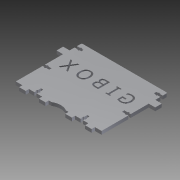
# Autodesk Inventor part: suport z darrera
Saved by Autodesk Inventor 2012 SP1 (Build 160190100, 190)
## iProperties
Created: 2015-03-29
Part Number: suport z darrera
Material: Default
Document SubType Name: Modeling
Designer: sheina
Density: 1 g/cm^3
Author: sheina
Autodesk Inventor part; units mm, degrees
ref_plane "YZ Plane" through (0, 0, 0) normal (1, 0, 0) x (0, 1, 0)
ref_plane "XZ Plane" through (0, 0, 0) normal (0, 1, 0) x (-1, 0, 0)
ref_plane "XY Plane" through (0, 0, 0) normal (0, 0, 1) x (1, 0, 0)
sketch "Boceto1" plane through (0, 0, 0) normal (0, 0, 1) x (1, 0, 0)
  line L0 (130, 0) -> (130, 95)
  line L1 (0, 95) -> (0, 0)
  line L2 (20, 0) -> (20, -5)
  line L3 (10, -5) -> (10, 0)
  line L4 (50, 0) -> (50, -5)
  line L5 (40, -5) -> (40, 0)
  line L6 (90, 0) -> (90, -5)
  line L7 (80, -5) -> (80, 0)
  line L8 (120, 0) -> (120, -5)
  line L9 (110, -5) -> (110, 0)
  line L10 (20, -5) -> (10, -5)
  line L11 (50, -5) -> (40, -5)
  line L12 (0, 0) -> (10, 0)
  line L13 (20, 0) -> (40, 0)
  line L14 (120, -5) -> (110, -5)
  line L15 (90, -5) -> (80, -5)
  line L16 (50, 0) -> (80, 0)
  line L17 (90, 0) -> (110, 0)
  line L18 (120, 0) -> (130, 0)
  line L19 (130, 100) -> (0, 100)
  line L20 (0, 95) -> (0, 100)
  line L21 (130, 95) -> (130, 100)
  dimension "d0" = 130
  dimension "d5" = 10
  dimension "d6" = 10
  dimension "d7" = 10
  dimension "d8" = 10
  dimension "d9" = 10
  dimension "d10" = 10
  dimension "d11" = 20
  dimension "d12" = 20
  constraints: 44 end point, 10 perpendicular, 7 parallel, 5 horizontal
  measures "d0" distance between parallel lines of L0 L1
  measures "d5" distance between parallel lines of L3 L2
  measures "d6" distance between parallel lines of L4 L5
  measures "d7" distance between parallel lines of L6 L7
  measures "d8" distance between parallel lines of L9 L8
  measures "d9" distance between parallel lines of L3 L1
  measures "d10" distance between parallel lines of L0 L8
  measures "d11" distance between parallel lines of L6 L9
  measures "d12" distance between parallel lines of L5 L2
extrude "Extrusión1" add sketch "Boceto1" along normal blind 5
sketch "Boceto2" plane through (0, 0, 5) normal (0, 0, 1) x (1, 0, 0)
  line L0 (80, 0) -> (50, 0) projected
  arc A0 (75.8724, 0) -> (54.3573, 0) centre (65.1148, -17.6132) ccw
  constraints: 2 point on circle, 2 point on line, 1 centre point
extrude "Extrusión2" cut sketch "Boceto2" against normal blind 5
sketch "Boceto3" plane through (0, 0, 5) normal (0, 0, 1) x (1, 0, 0)
  line L0 (80, -5) -> (80, 0) projected
  line L1 (40, 0) -> (20, 0) projected
  line L2 (98.3739, -0.0977) -> (98.3739, 2.6763)
  line L3 (98.3739, 2.6763) -> (97.3739, 2.6763)
  line L4 (97.3739, 2.6763) -> (97.3739, 5.0763)
  line L5 (97.3739, 5.0763) -> (98.3739, 5.0763)
  line L6 (98.3739, 5.0763) -> (98.3739, 9.9876)
  line L7 (98.3739, 9.9876) -> (101.8739, 9.9876)
  line L8 (101.8739, 9.9876) -> (101.8739, 5.0763)
  line L9 (101.8739, 5.0763) -> (102.8739, 5.0763)
  line L10 (102.8739, 5.0763) -> (102.8739, 2.6763)
  line L11 (102.8739, 2.6763) -> (101.8739, 2.6763)
  line L12 (101.8739, 2.6763) -> (101.8739, -0.0977)
  line L13 (28.1584, 5.0695) -> (28.1584, 9.9808)
  line L14 (31.6584, 9.9808) -> (31.6584, 5.0695)
  line L15 (28.1584, 9.9808) -> (31.6584, 9.9808)
  line L16 (27.1584, 5.0695) -> (28.1584, 5.0695)
  line L17 (28.1584, 2.6695) -> (27.1584, 2.6695)
  line L18 (27.1584, 2.6695) -> (27.1584, 5.0695)
  line L19 (31.6584, 2.6695) -> (31.6584, -0.1046)
  line L20 (28.1584, -0.1046) -> (28.1584, 2.6695)
  line L21 (32.6584, 2.6695) -> (31.6584, 2.6695)
  line L22 (32.6584, 5.0695) -> (32.6584, 2.6695)
  line L23 (31.6584, 5.0695) -> (32.6584, 5.0695)
  line L24 (28.1584, -0.1046) -> (31.6584, -0.1046)
  line L25 (98.3739, -0.0977) -> (101.8739, -0.0977)
  dimension "d18" = 3.5
  constraints: 48 end point, 3 parallel
  measures "d18" distance between parallel lines of L19 L20
extrude "Extrusión3" cut sketch "Boceto3" against normal blind 5
fillet "Empalme1" radius 2 2 edges at (130, 100, 2.5) (0, 100, 2.5)
sketch "Boceto5" plane through (0, 0, 0) normal (0, 0, -1) x (-1, 0, 0)
  line L0 (-115.5606, 70.7599) -> (-4.4465, 70.7599) construction
  line L1 (-4.4465, 70.7599) -> (-4.4465, 16.0729) construction
  line L2 (-4.4465, 16.0729) -> (-115.5606, 16.0729) construction
  line L3 (-115.5606, 16.0729) -> (-115.5606, 70.7599) construction
  spline S0 degree 2 poles (-106.196, 52.0306) (-108.1068, 52.0306) (-111.2721, 53.1975) (-112.4099, 54.379) knots 0 0 0 1 2 2 2
  spline S1 degree 2 poles (-112.4099, 54.379) (-113.5477, 55.5751) (-114.7584, 59.1051) (-114.7584, 61.3952) knots 0 0 0 1 2 2 2
  spline S2 degree 2 poles (-114.7584, 61.3952) (-114.7584, 63.5687) (-113.5331, 67.0111) (-112.3953, 68.2364) knots 0 0 0 1 2 2 2
  spline S3 degree 2 poles (-112.3953, 68.2364) (-111.3013, 69.4179) (-108.0922, 70.7016) (-106.1814, 70.7016) knots 0 0 0 1 2 2 2
  spline S4 degree 2 poles (-106.1814, 70.7016) (-105.2624, 70.7016) (-103.5995, 70.439) (-102.841, 70.2056) knots 0 0 0 1 2 2 2
  spline S5 degree 2 poles (-102.841, 70.2056) (-102.2284, 70.0306) (-100.7405, 69.3888) (-100.2884, 69.1554) knots 0 0 0 1 2 2 2
  line L4 (-100.2884, 69.1554) -> (-100.2884, 66.2672)
  line L5 (-100.2884, 66.2672) -> (-100.4926, 66.2672)
  spline S6 degree 2 poles (-100.4926, 66.2672) (-100.9448, 66.661) (-101.8929, 67.3758) (-102.7681, 67.7842) knots 0 0 0 1 2 2 2
  spline S7 degree 2 poles (-102.7681, 67.7842) (-103.4974, 68.1489) (-105.3791, 68.6302) (-106.4585, 68.6302) knots 0 0 0 1 2 2 2
  spline S8 degree 2 poles (-106.4585, 68.6302) (-109.055, 68.6302) (-112.264, 64.721) (-112.264, 61.4682) knots 0 0 0 1 2 2 2
  spline S9 degree 2 poles (-112.264, 61.4682) (-112.264, 59.6594) (-111.418, 56.9463) (-110.6157, 56.0127) knots 0 0 0 1 2 2 2
  spline S10 degree 2 poles (-110.6157, 56.0127) (-109.8427, 55.0792) (-107.6546, 54.1019) (-106.2835, 54.1019) knots 0 0 0 1 2 2 2
  spline S11 degree 2 poles (-106.2835, 54.1019) (-105.277, 54.1019) (-103.264, 54.3936) (-102.5785, 54.6853) knots 0 0 0 1 2 2 2
  line L6 (-102.5785, 54.6853) -> (-102.5785, 59.3385)
  line L7 (-102.5785, 59.3385) -> (-106.7503, 59.3385)
  line L8 (-106.7503, 59.3385) -> (-106.7503, 61.439)
  line L9 (-106.7503, 61.439) -> (-100.2154, 61.439)
  line L10 (-100.2154, 61.439) -> (-100.2154, 53.5768)
  spline S12 degree 2 poles (-100.2154, 53.5768) (-100.6676, 53.3725) (-102.2138, 52.7453) (-102.8702, 52.5557) knots 0 0 0 1 2 2 2
  spline S13 degree 2 poles (-102.8702, 52.5557) (-103.76, 52.2931) (-105.1895, 52.0306) (-106.196, 52.0306) knots 0 0 0 1 2 2 2
  line L11 (-83.2073, 52.3806) -> (-90.1798, 52.3806)
  line L12 (-90.1798, 52.3806) -> (-90.1798, 54.2186)
  line L13 (-90.1798, 54.2186) -> (-87.8897, 54.2186)
  line L14 (-87.8897, 54.2186) -> (-87.8897, 68.5427)
  line L15 (-87.8897, 68.5427) -> (-90.1798, 68.5427)
  line L16 (-90.1798, 68.5427) -> (-90.1798, 70.3806)
  line L17 (-90.1798, 70.3806) -> (-83.2073, 70.3806)
  line L18 (-83.2073, 70.3806) -> (-83.2073, 68.5427)
  line L19 (-83.2073, 68.5427) -> (-85.4974, 68.5427)
  line L20 (-85.4974, 68.5427) -> (-85.4974, 54.2186)
  line L21 (-85.4974, 54.2186) -> (-83.2073, 54.2186)
  line L22 (-83.2073, 54.2186) -> (-83.2073, 52.3806)
  spline S14 degree 2 poles (-60.3062, 57.909) (-60.3062, 56.567) (-61.3273, 54.5103) (-62.1733, 53.8393) knots 0 0 0 1 2 2 2
  spline S15 degree 2 poles (-62.1733, 53.8393) (-63.1944, 53.0516) (-65.5136, 52.3806) (-67.3516, 52.3806) knots 0 0 0 1 2 2 2
  line L23 (-67.3516, 52.3806) -> (-72.5153, 52.3806)
  line L24 (-72.5153, 52.3806) -> (-72.5153, 70.3806)
  line L25 (-72.5153, 70.3806) -> (-67.7454, 70.3806)
  spline S16 degree 2 poles (-67.7454, 70.3806) (-65.82, 70.3806) (-63.8945, 70.1327) (-63.0193, 69.6513) knots 0 0 0 1 2 2 2
  spline S17 degree 2 poles (-63.0193, 69.6513) (-62.042, 69.1408) (-61.1522, 67.4633) (-61.1522, 66.3255) knots 0 0 0 1 2 2 2
  spline S18 degree 2 poles (-61.1522, 66.3255) (-61.1522, 65.0565) (-62.4942, 63.0435) (-63.6757, 62.4747) knots 0 0 0 1 2 2 2
  line L26 (-63.6757, 62.4747) -> (-63.6757, 62.3871)
  spline S19 degree 2 poles (-63.6757, 62.3871) (-62.0712, 61.9495) (-60.3062, 59.6302) (-60.3062, 57.909) knots 0 0 0 1 2 2 2
  spline S20 degree 2 poles (-62.8005, 57.8069) (-62.8005, 58.828) (-63.384, 60.1408) (-64.2592, 60.6076) knots 0 0 0 1 2 2 2
  spline S21 degree 2 poles (-64.2592, 60.6076) (-64.8281, 60.8993) (-66.17, 61.0743) (-67.4099, 61.0743) knots 0 0 0 1 2 2 2
  line L27 (-67.4099, 61.0743) -> (-70.123, 61.0743)
  line L28 (-70.123, 61.0743) -> (-70.123, 54.4228)
  line L29 (-70.123, 54.4228) -> (-68.183, 54.4228)
  spline S22 degree 2 poles (-68.183, 54.4228) (-66.6076, 54.4228) (-64.7989, 54.7145) (-64.0987, 55.1813) knots 0 0 0 1 2 2 2
  spline S23 degree 2 poles (-64.0987, 55.1813) (-63.4277, 55.6627) (-62.8005, 56.8588) (-62.8005, 57.8069) knots 0 0 0 1 2 2 2
  spline S24 degree 2 poles (-63.6465, 65.99) (-63.6465, 66.6319) (-64.0841, 67.5946) (-64.5655, 67.8717) knots 0 0 0 1 2 2 2
  spline S25 degree 2 poles (-64.5655, 67.8717) (-65.149, 68.1926) (-66.5639, 68.3385) (-67.8329, 68.3385) knots 0 0 0 1 2 2 2
  line L30 (-67.8329, 68.3385) -> (-70.123, 68.3385)
  line L31 (-70.123, 68.3385) -> (-70.123, 63.0727)
  line L32 (-70.123, 63.0727) -> (-67.4099, 63.0727)
  spline S26 degree 2 poles (-67.4099, 63.0727) (-66.2867, 63.0727) (-65.2219, 63.3061) (-64.653, 63.6708) knots 0 0 0 1 2 2 2
  spline S27 degree 2 poles (-64.653, 63.6708) (-64.0987, 64.0208) (-63.6465, 65.144) (-63.6465, 65.99) knots 0 0 0 1 2 2 2
  spline S28 degree 2 poles (-37.4634, 68.3239) (-36.4423, 67.1278) (-35.3046, 63.627) (-35.3046, 61.3806) knots 0 0 0 1 2 2 2
  spline S29 degree 2 poles (-35.3046, 61.3806) (-35.3046, 59.1926) (-36.4132, 55.6481) (-37.4634, 54.452) knots 0 0 0 1 2 2 2
  spline S30 degree 2 poles (-37.4634, 54.452) (-38.572, 53.1975) (-41.5039, 52.0014) (-43.2689, 52.0014) knots 0 0 0 1 2 2 2
  spline S31 degree 2 poles (-43.2689, 52.0014) (-45.0922, 52.0014) (-48.0096, 53.2413) (-49.0744, 54.452) knots 0 0 0 1 2 2 2
  spline S32 degree 2 poles (-49.0744, 54.452) (-50.1101, 55.6481) (-51.2187, 59.1635) (-51.2187, 61.3806) knots 0 0 0 1 2 2 2
  spline S33 degree 2 poles (-51.2187, 61.3806) (-51.2187, 63.6416) (-50.0955, 67.0841) (-49.0598, 68.3239) knots 0 0 0 1 2 2 2
  spline S34 degree 2 poles (-49.0598, 68.3239) (-48.0096, 69.52) (-45.0777, 70.7599) (-43.2689, 70.7599) knots 0 0 0 1 2 2 2
  spline S35 degree 2 poles (-43.2689, 70.7599) (-41.431, 70.7599) (-38.4845, 69.4763) (-37.4634, 68.3239) knots 0 0 0 1 2 2 2
  spline S36 degree 2 poles (-37.7989, 61.3806) (-37.7989, 63.1602) (-38.572, 65.9171) (-39.2721, 66.8215) knots 0 0 0 1 2 2 2
  spline S37 degree 2 poles (-39.2721, 66.8215) (-39.9869, 67.755) (-41.9999, 68.6886) (-43.2543, 68.6886) knots 0 0 0 1 2 2 2
  spline S38 degree 2 poles (-43.2543, 68.6886) (-44.5525, 68.6886) (-46.5072, 67.7842) (-47.2511, 66.8215) knots 0 0 0 1 2 2 2
  spline S39 degree 2 poles (-47.2511, 66.8215) (-47.9658, 65.9025) (-48.7243, 63.1311) (-48.7243, 61.3806) knots 0 0 0 1 2 2 2
  spline S40 degree 2 poles (-48.7243, 61.3806) (-48.7243, 57.8361) (-45.7486, 54.0727) (-43.2543, 54.0727) knots 0 0 0 1 2 2 2
  spline S41 degree 2 poles (-43.2543, 54.0727) (-40.76, 54.0727) (-37.7989, 57.8361) (-37.7989, 61.3806) knots 0 0 0 1 2 2 2
  line L33 (-12.5055, 52.3806) -> (-15.2478, 52.3806)
  line L34 (-15.2478, 52.3806) -> (-19.6239, 59.5573)
  line L35 (-19.6239, 59.5573) -> (-24.0874, 52.3806)
  line L36 (-24.0874, 52.3806) -> (-26.6692, 52.3806)
  line L37 (-26.6692, 52.3806) -> (-20.9367, 61.3952)
  line L38 (-20.9367, 61.3952) -> (-26.4942, 70.3806)
  line L39 (-26.4942, 70.3806) -> (-23.7519, 70.3806)
  line L40 (-23.7519, 70.3806) -> (-19.4634, 63.3353)
  line L41 (-19.4634, 63.3353) -> (-15.0874, 70.3806)
  line L42 (-15.0874, 70.3806) -> (-12.5055, 70.3806)
  line L43 (-12.5055, 70.3806) -> (-18.136, 61.5119)
  line L44 (-18.136, 61.5119) -> (-12.5055, 52.3806)
  constraints: 2 other
extrude "Extrusión5" cut sketch "Boceto5" against normal blind 10
sketch "Boceto6" plane through (0, 0, 5) normal (0, 0, 1) x (1, 0, 0)
  line L0 (0, 0) -> (0, 100) projected
  line L1 (130, 100) -> (130, 0) projected
  line L2 (-9.8, 81.57) -> (-9.8, 71.57)
  line L3 (139.8, 71.57) -> (139.8, 81.57)
  line L4 (0, 71.57) -> (0, 81.57)
  line L5 (130, 81.57) -> (130, 71.57)
  line L6 (139.8, 81.57) -> (130, 81.57)
  line L7 (0, 81.57) -> (-9.8, 81.57)
  line L8 (-9.8, 71.57) -> (0, 71.57)
  line L9 (130, 71.57) -> (139.8, 71.57)
  point P0 (130, 93)
  point P1 (0, 93)
  dimension "d27" = 9.8
  dimension "d28" = 9.8
  constraints: 16 end point, 5 parallel, 4 point on line, 2 horizontal, 2 perpendicular
  measures "d27" distance between parallel lines of L0 L2
  measures "d28" distance between parallel lines of L1 L3
extrude "Extrusión6" add sketch "Boceto6" against normal blind 5
sketch "Boceto7" plane through (0, 0, 5) normal (0, 0, 1) x (1, 0, 0)
  line L0 (0, 0) -> (0, 71.57) projected
  line L1 (130.2524, 40.7442) -> (127.5829, 40.7442)
  line L2 (127.5829, 40.7442) -> (127.5829, 39.7442)
  line L3 (127.5829, 39.7442) -> (125.1829, 39.7442)
  line L4 (125.1829, 39.7442) -> (125.1829, 40.7442)
  line L5 (125.1829, 40.7442) -> (120.2716, 40.7442)
  line L6 (120.2716, 40.7442) -> (120.2716, 44.2442)
  line L7 (120.2716, 44.2442) -> (125.1829, 44.2442)
  line L8 (125.1829, 44.2442) -> (125.1829, 45.2442)
  line L9 (125.1829, 45.2442) -> (127.5829, 45.2442)
  line L10 (127.5829, 45.2442) -> (127.5829, 44.2442)
  line L11 (127.5829, 44.2442) -> (130.2524, 44.2442)
  line L12 (4.9356, 39.7466) -> (2.5356, 39.7466)
  line L13 (2.5356, 39.7466) -> (2.5356, 40.7466)
  line L14 (2.5356, 40.7466) -> (-0.1338, 40.7466)
  line L15 (4.9356, 40.7466) -> (4.9356, 39.7466)
  line L16 (9.8469, 40.7466) -> (4.9356, 40.7466)
  line L17 (-0.1338, 44.2466) -> (2.5356, 44.2466)
  line L18 (2.5356, 44.2466) -> (2.5356, 45.2466)
  line L19 (9.8469, 44.2466) -> (9.8469, 40.7466)
  line L20 (4.9356, 45.2466) -> (4.9356, 44.2466)
  line L21 (2.5356, 45.2466) -> (4.9356, 45.2466)
  line L22 (4.9356, 44.2466) -> (9.8469, 44.2466)
  line L23 (-0.1338, 40.7466) -> (-0.1338, 44.2466)
  line L24 (130.2524, 44.2442) -> (130.2524, 40.7442)
  constraints: 48 end point, 1 parallel
extrude "Extrusión7" cut sketch "Boceto7" against normal blind 10
sketch "Boceto8" plane through (0, 0, 0) normal (0, 0, -1) x (-1, 0, 0)
  line L0 (-130.3414, 92.7367) -> (-125.4301, 92.7367)
  line L1 (-130.3414, 89.2367) -> (-130.3414, 92.7367)
  line L2 (-125.4301, 89.2367) -> (-130.3414, 89.2367)
  line L3 (-125.4301, 92.7367) -> (-125.4301, 93.7367)
  line L4 (-123.0301, 93.7367) -> (-123.0301, 92.7367)
  line L5 (-123.0301, 92.7367) -> (-120.2561, 92.7367)
  line L6 (-120.2561, 89.2367) -> (-123.0301, 89.2367)
  line L7 (-125.4301, 88.2367) -> (-125.4301, 89.2367)
  line L8 (-123.0301, 88.2367) -> (-125.4301, 88.2367)
  line L9 (-123.0301, 89.2367) -> (-123.0301, 88.2367)
  line L10 (-120.2561, 89.2367) -> (-120.2561, 92.7367)
  line L11 (-125.4301, 93.7367) -> (-123.0301, 93.7367)
  line L12 (-4.8088, 88.2417) -> (-7.2088, 88.2417)
  line L13 (0.1025, 89.2417) -> (-4.8088, 89.2417)
  line L14 (0.1025, 92.7417) -> (0.1025, 89.2417)
  line L15 (-4.8088, 92.7417) -> (0.1025, 92.7417)
  line L16 (-7.2088, 92.7417) -> (-7.2088, 93.7417)
  line L17 (-9.9829, 92.7417) -> (-7.2088, 92.7417)
  line L18 (-9.9829, 92.7417) -> (-9.9829, 89.2417)
  line L19 (-7.2088, 93.7417) -> (-4.8088, 93.7417)
  line L20 (-4.8088, 93.7417) -> (-4.8088, 92.7417)
  line L21 (-7.2088, 89.2417) -> (-9.9829, 89.2417)
  line L22 (-4.8088, 89.2417) -> (-4.8088, 88.2417)
  line L23 (-7.2088, 88.2417) -> (-7.2088, 89.2417)
  dimension "d36" = 3.5
  dimension "d37" = 3.5
  constraints: 48 end point
  measures "d36" distance between parallel lines of L5 L6
  measures "d37" distance between parallel lines of L21 L17
extrude "Extrusión8" cut sketch "Boceto8" against normal blind 10
equation "\"d6\" = d5"
equation "\"d7\" = d5"
equation "\"d8\" = d5"
